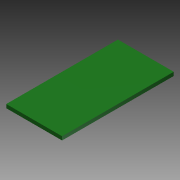
# Autodesk Inventor part: PeltierControllerBoard
Saved by Autodesk Inventor 2014 (Build 180170000, 170)
## iProperties
Created: 2015-04-19
Part Number: PeltierControllerBoard
Material: Generic
Document SubType Name: Modeling
Designer: Owner
Density: 1 g/cm^3
Appearance: Smooth - Dark Forest Green
Author: Owner
Autodesk Inventor part; units mm, degrees
ref_plane "YZ Plane" through (0, 0, 0) normal (1, 0, 0) x (0, 1, 0)
ref_plane "XZ Plane" through (0, 0, 0) normal (0, 1, 0) x (-1, 0, 0)
ref_plane "XY Plane" through (0, 0, 0) normal (0, 0, 1) x (1, 0, 0)
sketch "Sketch1" plane through (0, 0, 0) normal (0, 1, 0) x (-1, 0, 0)
  line L0 (-13.9872, 9.7538) -> (11.4128, 9.7538)
  line L1 (11.4128, 9.7538) -> (11.4128, -35.9662)
  line L2 (11.4128, -35.9662) -> (-13.9872, -35.9662)
  line L3 (-13.9872, -35.9662) -> (-13.9872, 9.7538)
  point P0 (0, 0)
  dimension "d0" = 25.4
  dimension "d1" = 45.72
  constraints: 8 end point, 2 parallel, 1 horizontal, 1 perpendicular
  measures "d0" distance of L0.start L0.end
  measures "d1" distance of L0.end L1.end
extrude "Extrusion1" add sketch "Sketch1" along normal blind 1.65
body "Solid1"
